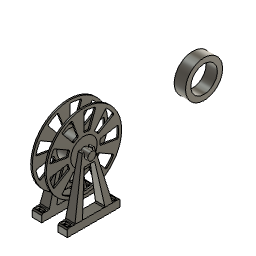
Strip Spool v8 (Autodesk Fusion 360 design; units mm, degrees)
Autodesk Fusion 360 part; units mm, degrees
sketch "Base" plane through (0, 0, 0) normal (1, 0, 0) x (0, 1, 0)
  circle A0 centre (0, 0) radius 35
  circle A1 centre (0, 0) radius 100
  circle A2 centre (0, 0) radius 11
  circle A3 centre (0, 0) radius 92
  line L0 (0, 43) -> (0, 92)
  line L1 (-14.7069, 40.4068) -> (-31.4659, 86.4517)
  line L2 (-27.6399, 32.9399) -> (-59.1365, 70.4761)
  line L3 (-37.2391, 21.5) -> (-79.6743, 46)
  line L4 (-42.3467, 7.4669) -> (-90.6023, 15.9756)
  line L5 (-42.3467, -7.4669) -> (-90.6023, -15.9756)
  line L6 (-37.2391, -21.5) -> (-79.6743, -46)
  line L7 (-27.6399, -32.9399) -> (-59.1365, -70.4761)
  line L8 (-14.7069, -40.4068) -> (-31.4659, -86.4517)
  line L9 (0, -43) -> (0, -92)
  line L10 (14.7069, -40.4068) -> (31.4659, -86.4517)
  line L11 (27.6399, -32.9399) -> (59.1365, -70.4761)
  line L12 (37.2391, -21.5) -> (79.6743, -46)
  line L13 (42.3467, -7.4669) -> (90.6023, -15.9756)
  line L14 (42.3467, 7.4669) -> (90.6023, 15.9756)
  line L15 (37.2391, 21.5) -> (79.6743, 46)
  line L16 (27.6399, 32.9399) -> (59.1365, 70.4761)
  line L17 (14.7069, 40.4068) -> (31.4659, 86.4517)
  circle A4 centre (0, 0) radius 43
  circle A5 centre (0, 0) radius 10.8
  line L18 (0, -100) -> (0, -150) construction
  dimension "d1" = 70
  dimension "d2" = 200
  dimension "d3" = 22
  dimension "d4" = -8
  dimension "d11" = 8
  dimension "d14" = -0.2
  dimension "d19" = 50
  constraint coincident A0.centre A1.centre
  constraint concentric A0 A1
  constraint coincident A3 L0.end
  constraint vertical L0
  constraint coincident A4 L1.start
  constraint coincident A4 L0.start
  constraint coincident A4 L17.start
  constraint coincident A4 L16.start
  constraint coincident A4 L15.start
  constraint coincident A4 L14.start
  constraint coincident A4 L13.start
  constraint coincident A4 L12.start
  constraint coincident A4 L11.start
  constraint coincident A4 L10.start
  constraint coincident A4 L9.start
  constraint coincident A4 L8.start
  constraint coincident A4 L7.start
  constraint coincident A4 L6.start
  constraint coincident A4 L5.start
  constraint coincident A4 L4.start
  constraint coincident A4 L3.start
  constraint coincident A4 L2.start
  constraint coincident A1 L18.start
  constraint vertical L18
  measures "d1" diameter of A0
  measures "d2" diameter of A1
  measures "d3" diameter of A2
  measures "d19" distance of L18.start L18.end
extrude "Extrude1" add sketch "Base" against normal blind 4 contours A1 | A3 L14 L15 A4 | A3 L12 L13 A4 | A4 | A3 L16 L17 A4 | A3 L10 L11 A4 | A3 L0 L1 A4 | A3 L8 L9 A4 | A3 L2 L3 A4 | A3 L6 L7 A4 | A3 L4 L5 A4 makes body 1
extrude "Extrude2" add sketch "Base" along normal blind 37 separate body contours A0 makes body 2
extrude "Extrude3" add sketch "Base" against normal blind 4 separate body contours A0 makes body 3
combine "Combine1" operation add target body 3 tool bodies 2
fillet "Fillet3" radius 2.5 36 edges at (-2, -79.6743, 46) (-2, -31.4659, 86.4517) (-2, 31.4659, 86.4517) (-2, -42.3467, 7.4669) (-2, -37.2391, -21.5) (-2, -42.3467, -7.4669) (-2, -37.2391, 21.5) (-2, -27.6399, 32.9399) (-2, -14.7069, 40.4068) (-2, 0, 43) (-2, 14.7069, 40.4068) (-2, 27.6399, 32.9399) (-2, 37.2391, 21.5) (-2, 42.3467, 7.4669) (-2, 42.3467, -7.4669) (-2, 37.2391, -21.5) (-2, 27.6399, -32.9399) (-2, 14.7069, -40.4068) (-2, 0, -43) (-2, -14.7069, -40.4068) (-2, -27.6399, -32.9399) (-2, -31.4659, -86.4517) (-2, -59.1365, -70.4761) (-2, 31.4659, -86.4517) (-2, 0, -92) (-2, 79.6743, -46) (-2, 59.1365, -70.4761) (-2, 90.6023, 15.9756) (-2, 90.6023, -15.9756) (-2, 59.1365, 70.4761) (-2, 79.6743, 46) (-2, 0, 92) (-2, -59.1365, 70.4761) (-2, -90.6023, 15.9756) (-2, -90.6023, -15.9756) (-2, -79.6743, -46) on bodies 1
copy_body "CopyPasteBodies1" bodies 1 makes body 4
move_body "Move1" bodies 4 to x (1, 0, 0) y (0, 1, 0) z (0, 0, 1) at (60, 0, 0)
move_body "Align1" bodies 4 to x (1, 0, 0) y (0, 1, 0) z (0, 0, 1) at (-23, 0, 0)
extrude "Extrude4" add sketch "Base" along normal blind -24 and the other way blind -58 separate body contours A5 makes body 5
sketch "Stand" plane through (0, 0, 0) normal (1, 0, 0) x (0, 1, 0)
  line L0 (0, -100) -> (0, -150)
  line L1 (0, -150) -> (-50, -150)
  line L2 (-50, -150) -> (0, -150)
  circle A0 centre (0, 0) radius 11
  line L3 (-11, 0) -> (-11, 12)
  line L4 (-11, 12) -> (-15, 12)
  line L5 (-15, 12) -> (-50, -130)
  line L6 (-50, -130) -> (-70, -130)
  line L7 (-70, -130) -> (-70, -150)
  line L8 (-70, -150) -> (-50, -150)
  line L9 (0, -11) -> (0, -150)
  arc A1 (-11, 0) -> (0, -11) centre (0, 0) ccw
  line L10 (0, -21.8062) -> (-13.9037, -21.8062)
  line L11 (-13.9037, -21.8062) -> (-30, -130)
  line L12 (-30, -130) -> (0, -130)
  constraint coincident L0.end L1.start
  constraint perpendicular L0 L1
  constraint coincident A0 L3.start
  constraint perpendicular L3 L4
  constraint perpendicular L3 L6
  constraint perpendicular L6 L7
  constraint perpendicular L3 L8
  constraint tangent L3 A1
  constraint coincident A0 L9.start
  constraint perpendicular L2 L9
  constraint coincident L9 L10.start
  constraint perpendicular L9 L10
  constraint coincident L9 L12.end
extrude "Extrude5" add sketch "Stand" against normal blind 25 from surface at -5 separate body contours L0 L1 L2 A0 L3 L4 L5 L6 L7 L8 L9 A1 L10 L11 L12 makes body 6
sketch "Slot" plane through (0, 0, -130) normal (0, 0, 1) x (-1, 0, 0)
  line L0 (5, 70) -> (5, 50)
  line L1 (5, 50) -> (30, 50)
  line L2 (30, 50) -> (30, 70)
  line L3 (30, 70) -> (5, 70)
  line L4 (23, 62) -> (12, 62)
  arc A0 (12, 62) -> (12, 58) centre (12, 60) ccw
  line L5 (12, 58) -> (23, 58)
  arc A1 (23, 58) -> (23, 62) centre (23, 60) ccw
  line L6 (25, 60) -> (10, 60) construction
  constraint tangent L4 A0
  constraint tangent A0 L5
  constraint parallel L4 L5
  constraint tangent L5 A1
  constraint tangent L4 A1
  constraint midpoint A1 L6.start
  constraint midpoint A0 L6.end
  constraint horizontal L6
extrude "Extrude6" cut sketch "Slot" against normal up to surface (20 mm away) contours L4 A0 L5 A1 bodies 6
chamfer "Chamfer1" distance 3 angle 45 4 edges at (-17.5, -58, -130) (-10, -60, -130) (-17.5, -62, -130) (-25, -60, -130) on bodies 6
chamfer "Chamfer2" distance 3 angle 45 1 edges at (-17.5, -70, -130) on bodies 6
mirror "Mirror1" about plane through (-5, 0, -130) normal (0, 1, 0) of bodies 6 merged
sketch "Sketch1" plane through (0, 0, 0) normal (1, 0, 0) x (0, 1, 0) in component "Spacer"
  circle A0 centre (325.9286, 0) radius 35.05
  circle A1 centre (325.9286, 0) radius 49.05
  dimension "d30" = 70.1
  dimension "d32" = 14
  measures "d30" diameter of A0
extrude "Extrude1'" add sketch "Sketch1" along normal blind 30 separate body makes body 7 in component "Spacer"
combine "Combine2" operation add target body 1 tool bodies 3
sketch "AngleCut" plane through (0, 0, 0) normal (0, 1, 0) x (1, 0, 0)
  line L0 (-5, -12) -> (-30, -12)
  line L1 (-30, 130) -> (-15, -12)
  line L2 (-56.0077, -12) -> (-56.0077, 130)
  line L3 (-56.0077, 130) -> (-30, 130)
  line L4 (-56.0077, -12) -> (-15, -12)
  constraint perpendicular L0 L2
  constraint perpendicular L2 L3
  constraint perpendicular L2 L4
  constraint coincident L0 L1.end
extrude "Extrude7" cut sketch "AngleCut" along normal mid plane 170 bodies 6
fillet "Fillet1" radius 2.5 10 edges at (-11.7855, -13.9037, -21.8062) (-11.7855, 13.9037, -21.8062) (-17.5, -30, -130) (-17.5, 30, -130) (-17.5, 50, -130) (-17.5, -50, -130) (-10, -15, 12) (-10, 15, 12) (-10, 11, 12) (-10, -11, 12) on bodies 6
ref_plane "WorkPlane1" through (16.5, 0, 0) normal (1, 0, 0) x (0, 1, 0)
mirror "Mirror2" about plane through (16.5, 0, 0) normal (1, 0, 0) of bodies 6 makes body 8
component "Spacer" placed x (1, 0, 0) y (0, 1, 0) z (0, 0, 1) at (0, 0, 0)
equation "d1 = CoreDiameter"
equation "d7 = -WallThikness"
equation "d9 = StipWidth + WallThikness + 3 mm"
equation "d12 = -WallThikness"
equation "d15 = -WallThikness - 20 mm"
equation "d17 = -WallThikness * 2 - StipWidth - 20 mm"
equation "CoreDiameter = 70 mm"
equation "d30 = CoreDiameter + 0.1 mm"
equation "SpacerOuterDiameter = 98 mm"
equation "d32 = ( SpacerOuterDiameter - CoreDiameter ) / 2"
equation "StipWidth = 30 mm"
equation "d34 = StipWidth"
equation "WallThikness = 4 mm"
equation "d41 = ( StipWidth + 3 mm ) / 2"
named bodies: "BaseCircle", "Inner", "Circle", "OuterCircle", "CenterPin", "Stand", "Stand Copy"
